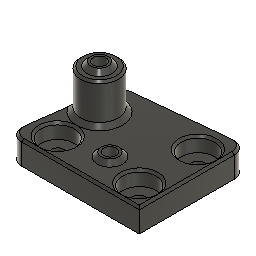
GT2_pulley_support_right_i2 v12 (Autodesk Fusion 360 design; units mm, degrees)
Autodesk Fusion 360 part; units mm, degrees
sketch "Sketch1" plane through (0, 0, 0) normal (0, 0, 1) x (1, 0, 0)
  circle A0 centre (-24.5, 5) radius 1.525
  circle A1 centre (-24.5, 5) radius 4
  circle A2 centre (-24.5, 15) radius 1.525
  circle A3 centre (-24.5, 15) radius 4.5
  line L0 (0, 0) -> (-31.5, 0)
  line L1 (-31.5, 0) -> (-31.5, 26)
  line L2 (-31.5, 26) -> (0, 26)
  line L3 (0, 26) -> (0, 0)
  circle A4 centre (-14, 7) radius 1.525
  circle A5 centre (-5, 5) radius 1.525
  circle A6 centre (-5, 5) radius 4
  circle A7 centre (-5, 19) radius 1.525
  circle A8 centre (-5, 19) radius 4
  line L4 (-16.7, 5.441154) -> (-14, 3.882309)
  line L5 (-14, 3.882309) -> (-11.3, 5.441154)
  line L6 (-11.3, 5.441154) -> (-11.3, 8.558846)
  line L7 (-11.3, 8.558846) -> (-14, 10.117692)
  line L8 (-14, 10.117692) -> (-16.7, 8.558846)
  line L9 (-16.7, 8.558846) -> (-16.7, 5.441154)
  line L10 (-21.8, 16.558846) -> (-24.5, 18.117691)
  line L11 (-24.5, 18.117691) -> (-27.2, 16.558846)
  line L12 (-27.2, 16.558846) -> (-27.2, 13.441154)
  line L13 (-27.2, 13.441154) -> (-24.5, 11.882309)
  line L14 (-24.5, 11.882309) -> (-21.8, 13.441154)
  line L15 (-21.8, 13.441154) -> (-21.8, 16.558846)
  line L16 (-31.5, 0) -> (-28.88601, 19.590943)
  line L17 (-31.5, 0) -> (-5.11345, 0) construction
  line L18 (0, 26) -> (-24.880294, 23.472752)
  line L19 (0, 26) -> (2, 26) construction
  arc A9 (-24.880294, 23.472752) -> (-28.88601, 19.590943) centre (-24.42554, 18.995789) ccw
  point P0 (-5, 19)
  point P1 (-14, 7)
  point P2 (-24.5, 15)
  dimension "d5" = 3.05
  dimension "d6" = 8
  dimension "d7" = 3.05
  dimension "d8" = 9
  dimension "d9" = 31.5
  dimension "d10" = 26
  dimension "d11" = 3.05
  dimension "d12" = 3.05
  dimension "d13" = 8
  dimension "d14" = 3.05
  dimension "d15" = 8
  dimension "d16" = 5
  dimension "d17" = 5
  dimension "d18" = 5
  dimension "d19" = 19
  dimension "d20" = 14
  dimension "d22" = 24.5
  dimension "d23" = 24.5
  dimension "d24" = 2.7
  dimension "d25" = 2.7
  dimension "d26" = 5
  dimension "d27" = 15
  dimension "d28" = 82.4
  dimension "d29" = 174.2
  dimension "d31" = 4.5
  dimension "d52" = 7
  constraint concentric A0 A1
  constraint concentric A2 A3
  constraint horizontal L0
  constraint vertical L1
  constraint horizontal L2
  constraint vertical L3
  constraint coincident L0.start L3.end
  constraint concentric A5 A6
  constraint concentric A7 A8
  constraint coincident P1 A4.centre
  constraint coincident P2 A2.centre
  constraint horizontal L17
  constraint horizontal L19
  constraint tangent L16 A9
  constraint tangent L18 A9
  measures "d5" diameter of A0
  measures "d6" diameter of A1
  measures "d7" diameter of A2
  measures "d8" diameter of A3
  measures "d9" distance of L0.start L0.end
  measures "d10" distance of L0.start L2.end
  measures "d11" diameter of A4
  measures "d12" diameter of A5
  measures "d13" diameter of A6
  measures "d14" diameter of A7
  measures "d15" diameter of A8
  measures "d16" horizontal distance of L0.start A5.centre
  measures "d17" vertical distance of L0.start A5.centre
  measures "d18" horizontal distance of P0 L0.start
  measures "d19" vertical distance of L0.start A7.centre
  measures "d20" horizontal distance of L0.start P1
  measures "d22" horizontal distance of L0.start A0.centre
  measures "d23" horizontal distance of L0.start P2
  measures "d24" distance of P1 L9
  measures "d25" distance of P2 L15
  measures "d26" vertical distance of L0.start A0.centre
  measures "d27" vertical distance of L0.start P2
  measures "d28" angle of L16 L17
  measures "d29" angle of L18 L19
  measures "d31" radius of A9
  measures "d52" vertical distance of L0.start P1
extrude "Extrude1" add sketch "Sketch1" along normal blind 15.5 contours A3 | L10 L11 L12 L13 L14 L15 picked at (-21.2, 15) picked at (-23.345833, 16.999075)
extrude "Extrude2" add sketch "Sketch1" along normal blind 6 contours L0 L3 L16 L18 A9 | L4 L5 L6 L7 L8 L9 picked at (-14.290851, 14.536454) picked at (-16.308333, 7)
extrude "Extrude3" add sketch "Sketch1" along normal blind 2.5 contours A1 | A6 | A8 picked at (-21.34557, 4.725514) picked at (-1.839892, 4.801277) picked at (-1.84557, 18.725514)
extrude "Extrude4" cut sketch "Sketch1" along normal blind 2.5 contours L4 L5 L6 L7 L8 L9 | L10 L11 L12 L13 L14 L15 picked at (-16.308333, 7) picked at (-23.345833, 16.999075)
fillet "Fillet1" radius 3 2 edges at (-31.5, 0, 3) (0, 26, 3)
sketch "Sketch2" plane through (0, 0, 15.5) normal (0, 0, 1) x (-1, 0, 0)
  circle A0 centre (24.5, -15) radius 1.525
  circle A1 centre (24.5, -15) radius 4.5
  circle A2 centre (24.5, -15) radius 2.05
  dimension "d41" = 4.1
  constraint concentric A0 A2
  measures "d41" diameter of A2
extrude "Extrude5" add sketch "Sketch2" along normal blind 1 contours A2 picked at (26.36169, -15.177609)
chamfer "Chamfer1" distance 1 angle 45 1 edges at (-22.588729, 14.258688, 15.5)
sketch "Sketch3" plane through (0, 0, 6) normal (0, 0, 1) x (-1, 0, 0)
  arc A0 (0, -22.679834) -> (3.303169, -25.664476) centre (3, -22.679834) ccw
  line L0 (3.303169, -25.664476) -> (24.880294, -23.472752)
  arc A1 (24.880294, -23.472752) -> (28.88601, -19.590943) centre (24.42554, -18.995789) ccw
  line L1 (28.88601, -19.590943) -> (31.046774, -3.396769)
  arc A2 (31.046774, -3.396769) -> (28.073128, 0) centre (28.073128, -3) ccw
  line L2 (28.073128, 0) -> (0, 0)
  line L3 (0, 0) -> (0, -22.679834)
  circle A3 centre (5, -5) radius 4
  circle A4 centre (5, -19) radius 4
  circle A5 centre (14, -7) radius 1.525
  circle A6 centre (24.5, -15) radius 4.5
  circle A7 centre (24.5, -5) radius 4
  circle A8 centre (14, -7) radius 2.05
  dimension "d45" = 4.1
  constraint concentric A5 A8
  measures "d45" diameter of A8
extrude "Extrude6" add sketch "Sketch3" along normal blind 1 contours A8 picked at (15.867368, -7.101846)
chamfer "Chamfer2" distance 1 angle 45 1 edges at (-12.088729, 6.258688, 6)
chamfer "Chamfer3" distance 0.5 angle 45 18 edges at (-28.229309, 6.446462, 6) (-8.729309, 6.446462, 6) (-8.729309, 20.446462, 6) (-28.695473, 13.372731, 15.5) (0, 11.339917, 6) (-0.98872, 24.905762, 6) (-14.091731, 24.568614, 6) (-27.557148, 22.227357, 6) (-29.966392, 11.493856, 6) (-30.330372, 1.023932, 6) (-14.036564, 0, 6) (-14.036564, 0, 0) (0, 11.339917, 0) (-0.98872, 24.905762, 0) (-14.091731, 24.568614, 0) (-27.557148, 22.227357, 0) (-29.966392, 11.493856, 0) (-30.330372, 1.023932, 0)
chamfer "Chamfer4" distance 1 angle 45 1 edges at (-20.03953, 14.404846, 6)
equation "d24 = ( 5.4 / 2 ) * 1 mm"
equation "d25 = ( 5.4 / 2 ) * 1 mm"
